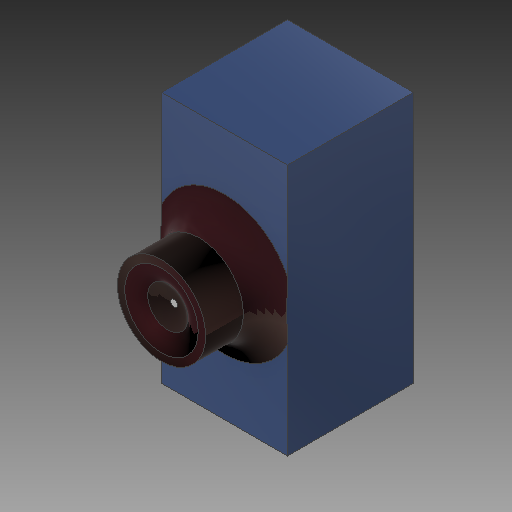
# Autodesk Inventor part: 红外
Saved by Autodesk Inventor 2017 (Build 210142000, 142)
## iProperties
Part Number: 红外
Material: 常规
Document SubType Name: Modeling
Designer: PANDA
Density: 1 g/cm^3
Appearance: 默认
Mass: 2.20487 g
Surface Area: 10.9557 cm^2
Volume: 2.20487 cm^3
Author: PANDA
Autodesk Inventor part; units mm, degrees
ref_plane "YZ Plane" through (0, 0, 0) normal (1, 0, 0) x (0, 1, 0)
ref_plane "XZ Plane" through (0, 0, 0) normal (0, 1, 0) x (-1, 0, 0)
ref_plane "XY Plane" through (0, 0, 0) normal (0, 0, 1) x (1, 0, 0)
sketch "草图1" plane through (0, 0, 0) normal (0, 1, 0) x (-1, 0, 0)
  line L0 (5, 5) -> (-5, 5)
  line L1 (-5, 5) -> (-5, -5)
  line L2 (-5, -5) -> (5, -5)
  line L3 (5, -5) -> (5, 5)
  point P0 (0, 0)
  dimension "d0" = 10
  dimension "d1" = 10
  constraints: 8 end point, 2 parallel, 1 horizontal, 1 perpendicular
  measures "d0" distance of L2.end L1.end
  measures "d1" distance of L1.end L0.end
extrude "拉伸1" add sketch "草图1" along normal blind 20
sketch "草图2" plane through (-5, 0, 5) normal (0, 0, 1) x (1, 0, 0)
  circle A0 centre (5, 10) radius 3.5
  point P0 (5, 0)
  dimension "d4" = 7
  constraints: 1 centre point
  measures "d4" diameter of A0
extrude "拉伸2" add sketch "草图2" along normal blind 5
sketch "草图3" plane through (0, 10, 10) normal (0, 0, 1) x (1, 0, 0)
  circle A0 centre (0, 0) radius 2
  point P0 (0, -10)
  dimension "d7" = 4
  constraints: 1 centre point
  measures "d7" diameter of A0
extrude "拉伸3" cut sketch "草图3" against normal blind 1
fillet "圆角1" radius 2 2 edges at (-3.5, 10, 5) (-2, 10, 9)
fillet "圆角2" radius 2 1 edges at (-2, 10, 10)
